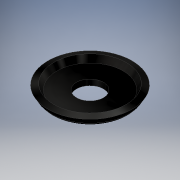
# Autodesk Inventor part: BottomBushingWasher
Saved by Autodesk Inventor 2019 (Build 230136000, 136)
## iProperties
Created: 2020-12-10
Part Number: BottomBushingWasher
Material: Aluminum
Document SubType Name: Modeling
Designer: Anass Hamdi
Density: 2.7 g/cm^3
Appearance: Aluminum Frame - Anodized Dark Bronze Satin
Author: Anass Hamdi
Autodesk Inventor part; units mm, degrees
ref_plane "YZ Plane" through (0, 0, 0) normal (1, 0, 0) x (0, 1, 0)
ref_plane "XZ Plane" through (0, 0, 0) normal (0, 1, 0) x (-1, 0, 0)
ref_plane "XY Plane" through (0, 0, 0) normal (0, 0, 1) x (1, 0, 0)
sketch "Sketch1" plane through (0, 0, 0) normal (0, 0, 1) x (1, 0, 0)
  line L0 (0, 0) -> (12.7, 0)
  line L1 (14.7, 0) -> (14.7, 3.5) construction
  line L2 (14.7, 3.5) -> (12.7, 3.5) construction
  line L3 (0, 0) -> (0, 2)
  line L4 (12.7, 3.5) -> (12.7, 4) construction
  line L5 (14.7, 3.5) -> (12.7, 4)
  line L6 (14.7, 3.5) -> (12.7, 0)
  line L7 (12.7, 4) -> (11.5571, 2)
  line L8 (0, 2) -> (11.5571, 2)
  dimension "d0" = 14.7
  dimension "d1" = 3.5
  dimension "d2" = 2
  dimension "d3" = 0.5
  dimension "d4" = 2
  dimension "d10" = 2
  constraints: 18 end point, 3 horizontal, 2 vertical, 1 parallel, 1 perpendicular
  measures "d0" distance of L0.start L1.start
  measures "d1" distance of L1.start L1.end
  measures "d2" distance of L1.end L2.end
  measures "d3" distance of L2.end L4.end
  measures "d4" distance of L0.start L3.end
  measures "d10" distance of L1.start L0.end
revolve "Revolution1" add sketch "Sketch1" angle 360 about axis through (0, 0, 0) along (0, 1, 0)
sketch "Sketch2" plane through (0, 2, 0) normal (0, 1, 0) x (1, 0, 0)
  circle A0 centre (0, 0) radius 4.7
  dimension "d6" = 9.4
  constraints: 1 centre point, 1 coincident
  measures "d6" diameter of A0
extrude "Extrusion1" cut sketch "Sketch2" against normal through all
fillet "Fillet1" radius 3 1 edges at (-12.7, 0, 0)
body "Solid1"
